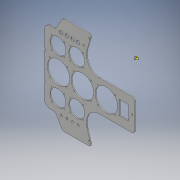
# Autodesk Inventor part: instrument_panel
Saved by Autodesk Inventor 2017.3 (Build 213256000, 256)
## iProperties
Created: 2017-11-25
Part Number: instrument_panel
Material: Generic
Document SubType Name: Modeling
Designer: Cedric
Density: 1 g/cm^3
Appearance: Default
Author: Cedric
Autodesk Inventor part; units mm, degrees
ref_plane "YZ Plane" through (0, 0, 0) normal (1, 0, 0) x (0, 1, 0)
ref_plane "XZ Plane" through (0, 0, 0) normal (0, 1, 0) x (-1, 0, 0)
ref_plane "XY Plane" through (0, 0, 0) normal (0, 0, 1) x (1, 0, 0)
sketch "Sketch1" plane through (0, 0, 0) normal (0, 1, 0) x (-1, 0, 0)
  line L0 (31.4392, 172.5) -> (-79.5, 172.5)
  line L1 (-34.5, -172.5) -> (31.4392, -172.5)
  line L2 (102.5, -107.5) -> (102.5, 107.5)
  line L3 (102.5, 172.5) -> (-102.5, -172.5) construction
  line L4 (-102.5, 172.5) -> (102.5, -172.5) construction
  line L5 (-132.5, 55) -> (-207.5, 55)
  line L6 (-217.5, 45) -> (-217.5, -45)
  line L7 (-217.5, -55) -> (-132.5, -55)
  line L8 (41.929, 166.3277) -> (60.071, 133.6723)
  line L9 (70.5608, 127.5) -> (82.5, 127.5)
  line L10 (102.5, 0) -> (-217.5, 0)
  line L11 (41.929, -166.3277) -> (60.071, -133.6723)
  line L12 (70.5608, -127.5) -> (82.5, -127.5)
  circle A0 centre (-208.1, 0) radius 3
  arc A1 (102.5, 107.5) -> (82.5, 127.5) centre (82.5, 107.5) ccw
  arc A2 (82.5, -127.5) -> (102.5, -107.5) centre (82.5, -107.5) ccw
  line L13 (-102.5, 149.5) -> (-102.5, 85)
  line L14 (-102.5, -85) -> (-102.5, -149.5)
  arc A3 (-132.5, 55) -> (-102.5, 85) centre (-132.5, 85) ccw
  arc A4 (-102.5, -85) -> (-132.5, -55) centre (-132.5, -85) ccw
  arc A5 (-79.5, 172.5) -> (-102.5, 149.5) centre (-79.5, 149.5) ccw
  arc A6 (-102.5, -149.5) -> (-79.5, -172.5) centre (-79.5, -149.5) ccw
  circle A7 centre (-55.1, -158) radius 3
  circle A8 centre (-55.1, 158) radius 3
  circle A9 centre (52.5, 0) radius 40
  circle A10 centre (83.489, 30.989) radius 1.85
  line L15 (52.5, 0) -> (83.489, 30.989)
  circle A11 centre (21.511, 30.989) radius 1.85
  circle A12 centre (21.511, -30.989) radius 1.85
  circle A13 centre (83.489, -30.989) radius 1.85
  circle A14 centre (-32.5, 0) radius 40
  circle A15 centre (-1.511, 30.989) radius 1.85
  line L16 (-32.5, 0) -> (-1.511, 30.989)
  circle A16 centre (-63.489, 30.989) radius 1.85
  circle A17 centre (-63.489, -30.989) radius 1.85
  circle A18 centre (-1.511, -30.989) radius 1.85
  circle A19 centre (-117.5, 0) radius 40
  circle A20 centre (-86.511, 30.989) radius 1.85
  line L17 (-117.5, 0) -> (-86.511, 30.989)
  circle A21 centre (-148.489, 30.989) radius 1.85
  circle A22 centre (-148.489, -30.989) radius 1.85
  circle A23 centre (-86.511, -30.989) radius 1.85
  circle A24 centre (54.5, 80) radius 28.5
  line L18 (54.5, 80) -> (83, 80)
  line L19 (54.5, 80) -> (74.6525, 100.1525)
  circle A25 centre (77.3749, 102.8749) radius 1.85
  circle A26 centre (31.6251, 102.8749) radius 1.85
  circle A27 centre (31.6251, 57.1251) radius 1.85
  circle A28 centre (77.3749, 57.1251) radius 1.85
  circle A29 centre (-12.5, 80) radius 28.5
  line L20 (-12.5, 80) -> (16, 80)
  line L21 (-12.5, 80) -> (7.6525, 100.1525)
  circle A30 centre (10.3749, 102.8749) radius 1.85
  circle A31 centre (-35.3749, 102.8749) radius 1.85
  circle A32 centre (-35.3749, 57.1251) radius 1.85
  circle A33 centre (10.3749, 57.1251) radius 1.85
  circle A34 centre (54.5, -80) radius 28.5
  line L22 (54.5, -80) -> (83, -80)
  line L23 (54.5, -80) -> (74.6525, -59.8475)
  circle A35 centre (77.3749, -57.1251) radius 1.85
  circle A36 centre (31.6251, -57.1251) radius 1.85
  circle A37 centre (31.6251, -102.8749) radius 1.85
  circle A38 centre (77.3749, -102.8749) radius 1.85
  circle A39 centre (-12.5, -80) radius 28.5
  line L24 (-12.5, -80) -> (16, -80)
  line L25 (-12.5, -80) -> (7.6525, -59.8475)
  circle A40 centre (10.3749, -57.1251) radius 1.85
  circle A41 centre (-35.3749, -57.1251) radius 1.85
  circle A42 centre (-35.3749, -102.8749) radius 1.85
  circle A43 centre (10.3749, -102.8749) radius 1.85
  line L26 (-197, -25) -> (-163, -25)
  line L27 (-163, -25) -> (-163, 25)
  line L28 (-163, 25) -> (-197, 25)
  line L29 (-197, 25) -> (-197, -25)
  line L30 (-197, -25) -> (-163, 25) construction
  line L31 (-163, -25) -> (-197, 25) construction
  circle A44 centre (-17.5, 127.5) radius 6
  circle A45 centre (2.5, 127.5) radius 6
  circle A46 centre (22.5, 127.5) radius 6
  circle A47 centre (42.5, 127.5) radius 6
  line L32 (-79.5, -127.5) -> (-79.5, -100)
  line L33 (-124.5, -55) -> (-217.5, -55)
  line L34 (-79.5, -172.5) -> (31.4392, -172.5)
  arc A48 (-79.5, -100) -> (-124.5, -55) centre (-124.5, -100) ccw
  arc A49 (-79.5, -127.5) -> (-34.5, -172.5) centre (-34.5, -127.5) ccw
  line L35 (-34.5, 172.5) -> (31.4392, 172.5)
  line L36 (-79.5, 127.5) -> (-79.5, 100)
  line L37 (-124.5, 55) -> (-217.5, 55)
  arc A50 (-124.5, 55) -> (-79.5, 100) centre (-124.5, 100) ccw
  arc A51 (-34.5, 172.5) -> (-79.5, 127.5) centre (-34.5, 127.5) ccw
  arc A52 (31.4392, -172.5) -> (41.929, -166.3277) centre (31.4392, -160.5) ccw
  arc A53 (41.929, 166.3277) -> (31.4392, 172.5) centre (31.4392, 160.5) ccw
  arc A54 (70.5608, -127.5) -> (60.071, -133.6723) centre (70.5608, -139.5) ccw
  arc A55 (60.071, 133.6723) -> (70.5608, 127.5) centre (70.5608, 139.5) ccw
  line L38 (-47.5, -115.6878) -> (-47.5, -100)
  line L39 (-92.5, -55) -> (-207.5, -55)
  line L40 (-47.5, -172.5) -> (31.4392, -172.5)
  line L41 (-48.0352, -119.2314) -> (-61.6974, -163.4329)
  arc A56 (-47.5, -100) -> (-92.5, -55) centre (-92.5, -100) ccw
  arc A57 (-48.0352, -119.2314) -> (-47.5, -115.6878) centre (-59.5, -115.6878) ccw
  line L42 (-55.0096, -172.5) -> (31.4392, -172.5)
  arc A58 (-61.6974, -163.4329) -> (-55.0096, -172.5) centre (-55.0096, -165.5) ccw
  line L43 (-47.5, 115.6878) -> (-47.5, 100)
  line L44 (-92.5, 55) -> (-217.5, 55)
  line L45 (-48.0352, 119.2314) -> (-61.6974, 163.4329)
  arc A59 (-92.5, 55) -> (-47.5, 100) centre (-92.5, 100) ccw
  arc A60 (-47.5, 115.6878) -> (-48.0352, 119.2314) centre (-59.5, 115.6878) ccw
  line L46 (-55.0096, 172.5) -> (31.4392, 172.5)
  arc A61 (-55.0096, 172.5) -> (-61.6974, 163.4329) centre (-55.0096, 165.5) ccw
  circle A62 centre (102.5, 46) radius 4
  circle A63 centre (102.5, -49) radius 3
  circle A64 centre (-37.5, 127.5) radius 3.5
  arc A65 (-217.5, -45) -> (-207.5, -55) centre (-207.5, -45) ccw
  arc A66 (-207.5, 55) -> (-217.5, 45) centre (-207.5, 45) ccw
  circle A67 centre (42.5, -127.5) radius 3.5
  circle A68 centre (22.5, -127.5) radius 3.5
  circle A69 centre (2.5, -127.5) radius 3.5
  circle A70 centre (-17.5, -127.5) radius 3.5
  line L47 (-124.5, 55) -> (-132.5, 55)
  line L48 (-34.5, 172.5) -> (-79.5, 172.5)
  arc A71 (-61.6767, 163.3668) -> (-61.6974, 163.4329) centre (-55.0096, 165.5) ccw
  arc A72 (-61.6767, 163.3668) -> (-79.5, 127.5) centre (-34.5, 127.5) ccw
  line L49 (-79.5, 127.5) -> (-79.5, 100)
  line L50 (-61.6974, 163.4329) -> (-47.6345, 117.4797)
  line L51 (-47.5, 100) -> (-47.6345, 117.4797)
  line L52 (-92.5, 55) -> (-124.5, 55)
  line L53 (-92.5, 55) -> (-124.5, 55)
  line L54 (-92.5, 55) -> (-124.5, 55)
  line L55 (-55.0096, 172.5) -> (-79.5, 172.5)
  line L56 (-34.5, 172.5) -> (-55.0096, 172.5)
  arc A73 (-34.5, 172.5) -> (-61.6771, 163.3665) centre (-34.5, 127.5) ccw
  arc A74 (-55.0096, 172.5) -> (-61.6766, 163.3666) centre (-55.0096, 165.5) ccw
  point P0 (0, 0)
  point P1 (-102.5, 55)
  point P2 (63.5, 127.5)
  point P3 (38.5, 172.5)
  point P4 (102.5, 127.5)
  point P5 (63.5, -127.5)
  point P6 (38.5, -172.5)
  point P7 (102.5, -127.5)
  point P8 (-102.5, -55)
  point P9 (-12.5, 101)
  point P10 (69.5, -67.7951)
  point P11 (-13.8374, -72.5218)
  point P12 (-180, 0)
  point P13 (-47.5, -117.5)
  point P14 (-64.5, -172.5)
  dimension "d0" = 345
  dimension "d1" = 205
  dimension "d2" = 110
  dimension "d4" = 55
  dimension "d5" = 141
  dimension "d6" = 45
  dimension "d7" = 25
  dimension "d8" = 172.5
  dimension "d9" = 102.5
  dimension "d10" = 320
  dimension "d11" = 9.4
  dimension "d12" = 6
  dimension "d13" = 20
  dimension "d14" = 20
  dimension "d15" = 115
  dimension "d16" = 115
  dimension "d17" = 30
  dimension "d18" = 23
  dimension "d19" = 153
  dimension "d20" = 158
  dimension "d21" = 6
  dimension "d22" = 80
  dimension "d23" = 3.7
  dimension "d24" = 43.825
  dimension "d25" = 45
  dimension "d28" = 360
  dimension "d30" = 50
  dimension "d33" = 80
  dimension "d34" = 3.7
  dimension "d35" = 43.825
  dimension "d36" = 360
  dimension "d41" = 80
  dimension "d42" = 3.7
  dimension "d43" = 43.825
  dimension "d44" = 360
  dimension "d45" = 135
  dimension "d46" = 220
  dimension "d50" = 45
  dimension "d51" = 85
  dimension "d52" = 85
  dimension "d53" = 57
  dimension "d54" = 45
  dimension "d55" = 3.7
  dimension "d56" = 3.85
  dimension "d59" = 360
  dimension "d61" = 80
  dimension "d62" = 48
  dimension "d71" = 57
  dimension "d72" = 45
  dimension "d73" = 3.7
  dimension "d74" = 3.85
  dimension "d75" = 360
  dimension "d86" = 57
  dimension "d87" = 45
  dimension "d88" = 3.7
  dimension "d89" = 3.85
  dimension "d90" = 360
  dimension "d103" = 57
  dimension "d104" = 45
  dimension "d105" = 3.7
  dimension "d106" = 3.85
  dimension "d107" = 360
  dimension "d108" = 115
  dimension "d109" = 115
  constraints: 114 end point, 75 centre point, 62 point on circle, 45 tangent, 43 point on line, 23 symmetric about line, 11 collinear, 8 horizontal, 7 coincident, 7 parallel, 6 midpoint, 6 perpendicular, 5 equal radius, 1 vertical, 69 other
  measures "d0" distance of L4.end L3.start
  measures "d1" distance of L3.end L4.end
  measures "d2" distance of L37.end L7.start
  measures "d4" distance from line of point (0, 0) L7
  measures "d5" distance of point (38.5, 172.5) L4.start
  measures "d6" vertical distance of point (38.5, 172.5) point (63.5, 127.5)
  measures "d7" horizontal distance of point (38.5, 172.5) point (63.5, 127.5)
  measures "d8" distance from line of point (0, 0) L0
  measures "d9" distance from line of L2 point (0, 0)
  measures "d10" distance of L10.start L10.end
  measures "d11" distance from line of L6 A0.centre
  measures "d12" diameter of A0
  measures "d13" radius of A1
  measures "d14" radius of A2
  measures "d15" distance from line of L6 point (-102.5, 55)
  measures "d16" distance of point (-102.5, -55) L7.start
  measures "d17" radius of A3
  measures "d18" radius of A5
  measures "d19" horizontal distance of A0.centre A7.centre
  measures "d20" vertical distance of A0.centre A7.centre
  measures "d21" diameter of A7
  measures "d22" diameter of A9
  measures "d23" diameter of A10
  measures "d24" distance of L15.end L15.start
  measures "d25" angle of L15 L10
  measures "d30" distance from line of L15.start L2
  measures "d33" diameter of A14
  measures "d34" diameter of A15
  measures "d35" distance of L16.end L16.start
  measures "d41" diameter of A19
  measures "d42" diameter of A20
  measures "d43" distance of L17.end L17.start
  measures "d45" distance from line of L2 L16.start
  measures "d46" distance from line of L2 L17.start
  measures "d50" angle of L16 L10
  measures "d51" distance of L17.start L16.start
  measures "d52" distance of L16.start L15.start
  measures "d53" diameter of A24
  measures "d54" angle of L19 L18
  measures "d55" diameter of A25
  measures "d56" distance of A25.centre L19.end
  measures "d61" vertical distance of L18.start L15.start
  measures "d62" distance from line of L2 L18.start
  measures "d71" diameter of A29
  measures "d72" angle of L21 L20
  measures "d73" diameter of A30
  measures "d74" distance of A30.centre L21.end
  measures "d86" diameter of A34
  measures "d87" angle of L23 L22
  measures "d88" diameter of A35
  measures "d89" distance of A35.centre L23.end
  measures "d103" diameter of A39
  measures "d104" angle of L25 L24
  measures "d105" diameter of A40
  measures "d106" distance of A40.centre L25.end
  measures "d108" distance from line of L2 L20.start
  measures "d109" distance from line of L2 L24.start
extrude "Extrusion1" add sketch "Sketch1" along normal blind 3 contours A53 L8 A55 L9 A1 L2 A62 L10 A9 A14 A19 L27 L28 L29 A0 L6 A66 L5 L37 L44 A59 L43 A60 L45 A71 A8 A51 L0 | A51 A71 A61 L0 | A61 L45 A51 L36 A50 L37 A3 L13 A5 L0 | A71 A8 A51 | A51 L45 A71 | L50 L51 A59 L44 A50 L36 A51 | L45 A60 L50 | A60 L43 L51 | L2 A62 | L2 A63 A2 L12 A54 L11 A52 L1 A49 L41 A57 L38 A56 L39 L33 L7 A65 L6 L10 A0 L29 L26 L27 A19 A14 A9 | L2 A63 | A9 L10 | L10 L15 A9 | A0 L10 | L10 A0 | L10 A9 L15 | A14 L10 | L10 L16 A14 | L29 L28 L27 L10 | L10 L27 L26 L29 | L10 A14 L16 | A19 L10 | L10 L17 A19 | A19 L17 L10 | A58 L41 A49 L34 picked at (102.1809, 47.2946) picked at (101.5073, -49.1205)
extrude "Extrusion2" cut sketch "Sketch1" along normal blind 3 contours A9 L10 | L10 L15 A9 | L10 A9 L15 | A14 L10 | L10 L16 A14 | L29 L28 L27 L10 | L10 L27 L26 L29 | L10 A14 L16 | A19 L10 | L10 L17 A19 | A19 L17 L10
extrude "Extrusion3" cut sketch "Sketch1" along normal blind 3 contours A62 L2 | L2 A62 | A63 L2 | L2 A63
extrude "Extrusion4" cut sketch "Sketch1" along normal blind 3 contours A0 L10 | L10 A0
extrude "Extrusion12" cut sketch "Sketch1" along normal blind 10 contours A51 A71 A61 L0 | A61 L45 A51 L36 A50 L37 A3 L13 A5 L0 | A51 L45 A71 | L50 L51 A59 L44 A50 L36 A51
extrude "Extrusion13" add sketch "Sketch1" along normal blind 3 contours A51 A71 A61 L0 | A51 L45 A71
equation "\"d4\" = 0.5 * d2"
equation "\"d8\" = 0.5 * d0"
equation "\"d9\" = 0.5 * d1"
equation "\"d16\" = d15"
body "Solid2"
